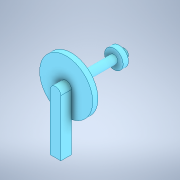
# Autodesk Inventor part: outerGear
Saved by Autodesk Inventor 2020.1 (Build 241239000, 239)
## iProperties
Created: 2020-01-18
Part Number: outerGear
Material: Generic
Document SubType Name: Modeling
Designer: Ali
Density: 1 g/cm^3
Appearance: Default
Author: Ali
Autodesk Inventor part; units mm, degrees
ref_plane "YZ Plane" through (0, 0, 0) normal (1, 0, 0) x (0, 1, 0)
ref_plane "XZ Plane" through (0, 0, 0) normal (0, 1, 0) x (-1, 0, 0)
ref_plane "XY Plane" through (0, 0, 0) normal (0, 0, 1) x (1, 0, 0)
sketch "Sketch1" plane through (0, 0, 0) normal (0, 0, 1) x (1, 0, 0)
  circle A0 centre (0, 0) radius 5
  dimension "d0" = 10
  constraints: 1 centre point, 1 coincident
  measures "d0" diameter of A0
extrude "Extrusion1" add sketch "Sketch1" along normal blind 1
sketch "Sketch2" plane through (0, 0, 1) normal (0, 0, 1) x (1, 0, 0)
  circle A0 centre (0, 0) radius 0.75
  dimension "d3" = 1.5
  constraints: 1 centre point, 1 coincident
  measures "d3" diameter of A0
extrude "Extrusion2" add sketch "Sketch2" along normal blind 10
sketch "Sketch3" plane through (0, 0, 0) normal (0, 0, -1) x (-1, 0, 0)
  circle A0 centre (0, 0) radius 0.75 projected
  circle A1 centre (0, 0) radius 1
  dimension "d6" = 2
  constraints: 1 centre point, 1 coincident
  measures "d6" diameter of A1
extrude "Extrusion3" add sketch "Sketch3" along normal blind 2
sketch "Sketch4" plane through (0, 0, -2) normal (0, 0, -1) x (-1, 0, 0)
  circle A0 centre (0, 0) radius 1 projected
  circle A1 centre (0, 0) radius 1 construction
  line L0 (-1, 0) -> (1, 0) construction
  line L1 (-1, 0) -> (1, 0)
  line L2 (1, 0) -> (1, -10.6446)
  line L3 (1, -10.6446) -> (-1, -10.6446)
  line L4 (-1, -10.6446) -> (-1, 0)
  point P0 (1, 0)
  point P1 (-1, 0)
  dimension "d9" = 2
  dimension "d10" = 10.6446
  constraints: 10 end point, 2 horizontal, 2 parallel, 2 point on circle, 1 perpendicular
  measures "d9" distance between parallel lines of L4 L2
  measures "d10" distance of L1.end L2.end
extrude "Extrusion4" add sketch "Sketch4" against normal blind 2 contours L2 L3 L4 A0
extrude "Extrusion6" add sketch "Sketch3" along normal blind 2 contours A0
ref_plane "Work Plane1" through (0, 0, 10) normal (0, 0, 1) x (1, 0, 0)
sketch "Sketch5" plane through (0, 0, 10) normal (0, 0, 1) x (1, 0, 0)
  circle A0 centre (0, 0) radius 0.75 projected
  circle A1 centre (0, 0) radius 1.75
  dimension "d18" = 1
  constraints: 1 centre point
  measures "d18" radial gap between concentric circles of A0 A1
extrude "Extrusion7" add sketch "Sketch5" against normal blind 1
equation "\"d0\" = OG_gearDiameter"
equation "\"d1\" = OG_gearThickness"
equation "\"d3\" = OG_shaftDiameter"
equation "\"d4\" = OG_shaftLength"
equation "\"d6\" = LE_baseDiameter"
equation "\"d7\" = LE_thickness"
equation "\"d9\" = LE_thickness"
equation "\"d10\" = LE_maxLength"
equation "\"d11\" = LE_thickness"
equation "\"d15\" = LE_thickness + LE_offsetAboveOuterGear"
equation "\"d18\" = OG_skirtOffset"
equation "\"d19\" = OG_skirtThickness"
equation "\"Wheel_Related_W_\" = 0"
equation "\"W_innerDiameter\" = 35"
equation "\"W_innerDepth\" = 5"
equation "\"W_wallThickness\" = 1"
equation "\"W_holesClearance\" = 0.1"
equation "\"W_outerGearHoleDiameter\" = 1.7"
equation "\"W_innerGearHoleDiameter\" = 4.7"
equation "\"TempSpotReserved7\" = 0"
equation "\"TempSpotReserved8\" = 0"
equation "\"TempSpotReserved9\" = 0"
equation "\"TempSpotReserved10\" = 0"
equation "\"TempSpotReserved11\" = 0"
equation "\"TempSpotReserved12\" = 0"
equation "\"TempSpotReserved13\" = 0"
equation "\"TempSpotReserved14\" = 0"
equation "\"TempSpotReserved15\" = 0"
equation "\"TempSpotReserved16\" = 0"
equation "\"TempSpotReserved17\" = 0"
equation "\"TempSpotReserved18\" = 0"
equation "\"TempSpotReserved19\" = 0"
equation "\"TempSpotReserved20\" = 0"
equation "\"Inner_Gear_Related_IG_\" = 0"
equation "\"IG_shaftDiameter\" = 2.5"
equation "\"IG_shaftLength\" = 15"
equation "\"IG_gearThickness\" = 1"
equation "\"TempSpotReserved25\" = 0"
equation "\"TempSpotReserved26\" = 0"
equation "\"TempSpotReserved27\" = 0"
equation "\"TempSpotReserved28\" = 0"
equation "\"TempSpotReserved29\" = 0"
equation "\"TempSpotReserved30\" = 0"
equation "\"TempSpotReserved31\" = 0"
equation "\"TempSpotReserved32\" = 0"
equation "\"TempSpotReserved33\" = 0"
equation "\"TempSpotReserved34\" = 0"
equation "\"TempSpotReserved35\" = 0"
equation "\"TempSpotReserved36\" = 0"
equation "\"TempSpotReserved37\" = 0"
equation "\"TempSpotReserved38\" = 0"
equation "\"TempSpotReserved39\" = 0"
equation "\"TempSpotReserved40\" = 0"
equation "\"Outer_Gear_Related_OG_\" = 0"
equation "\"OG_shaftDiameter\" = 1.5"
equation "\"OG_gearDiameter\" = 10"
equation "\"OG_shaftLength\" = 10"
equation "\"OG_gearThickness\" = 1"
equation "\"TempSpotReserved47\" = 0"
equation "\"TempSpotReserved48\" = 0"
equation "\"TempSpotReserved49\" = 0"
equation "\"TempSpotReserved50\" = 0"
equation "\"TempSpotReserved51\" = 0"
equation "\"TempSpotReserved52\" = 0"
equation "\"TempSpotReserved53\" = 0"
equation "\"TempSpotReserved54\" = 0"
equation "\"TempSpotReserved55\" = 0"
equation "\"TempSpotReserved56\" = 0"
equation "\"TempSpotReserved57\" = 0"
equation "\"TempSpotReserved58\" = 0"
equation "\"TempSpotReserved59\" = 0"
equation "\"TempSpotReserved60\" = 0"
equation "\"Leg_Extensions_Related_LE_\" = 0"
equation "\"LE_baseDiameter\" = 2"
equation "\"LE_maxLength\" = 10.64459"
equation "\"LE_thickness\" = 2"
equation "\"B_bearingThickness\" = 1"
equation "\"TempSpotReserved43\" = 0"
equation "\"TempSpotReserved45\" = 0"
equation "\"Thisisatest\" = 25.4"
equation "\"TempSpotReserved46\" = 0"
equation "\"TempSpotReserved44\" = 0"
equation "\"LE_offsetAboveOuterGear\" = 0"
equation "\"Bearing_Related_B_\" = 0"
equation "\"TempSpotReserved42\" = 0"
equation "\"d17\" = -W_wallThickness"
equation "\"OG_skirtOffset\" = 1"
equation "\"OG_skirtThickness\" = 1"
equation "\"IG_skirtThickness\" = 0.5"
equation "\"IG_skirtOffset\" = 1.5"
body "Solid1"
